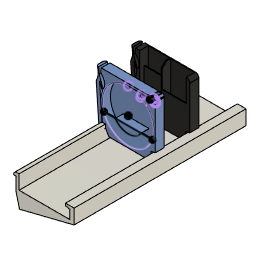
SMD Cassette System v11 (Autodesk Fusion 360 design; units mm, degrees)
Autodesk Fusion 360 part; units mm, degrees
note: some values were not read from the file. Set by a fixed rule: which face or edge a step refers to.
sketch "Base Shape" plane through (0, 0, 0) normal (0, 1, 0) x (1, 0, 0)
  line L0 (5, -7) -> (5, -11)
  line L1 (5, -11) -> (0, -11)
  line L2 (0, -65) -> (0, -11)
  line L3 (63, -65) -> (0, -65)
  line L4 (63, -11) -> (63, -65)
  line L5 (58, -10.01) -> (63, -11)
  line L6 (58, -4.99) -> (58, -10.01)
  line L7 (63, -4) -> (58, -4.99)
  line L8 (9, 0) -> (5, -7)
  line L9 (59.0007, 0) -> (9, 0)
  line L10 (63, -7.5) -> (58, -7.5) construction
  arc A0 (63, -4) -> (59.0007, 0) centre (59.0007, -3.9993) ccw
  line L11 (0, -1.75) -> (0, -22.5) construction
  line L12 (1.75, 0) -> (22.5, 0) construction
  line L13 (0.3, -10.5) -> (4.5, -10.5)
  line L14 (4.5, -10.5) -> (4.5, 6)
  line L15 (4.5, 6) -> (63.5, 6)
  line L16 (63.5, 6) -> (63.5, -4.41)
  line L17 (63.5, -4.41) -> (58.5, -5.4)
  line L18 (58.5, -5.4) -> (58.5, -8)
  line L19 (68.5, -8) -> (68.5, 9)
  line L20 (68.5, 9) -> (4.9505, 24.8447)
  line L21 (1, 9) -> (1, -6.5)
  line L22 (-1.7, -8.5) -> (-1.7, -6.5)
  line L23 (1, -6.5) -> (-1.7, -6.5)
  line L24 (68.5, 9) -> (1, 9)
  line L25 (1, 9) -> (4.9505, 24.8447)
  line L26 (0.3, -10.5) -> (-1.7, -8.5)
  line L27 (58.5, -8) -> (68.5, -8)
  line L28 (0.3, -10.5) -> (0.3, -8.5) construction
  line L29 (0.3, -8.5) -> (-1.7, -8.5) construction
  line L30 (31.5, -65) -> (31.5, 6) construction
  dimension "d139" = 4
  dimension "d140" = 7
  dimension "d141" = 65
  dimension "d142" = 63
  dimension "d144" = 4
  dimension "d168" = 7
  dimension "d216" = 3.5
  dimension "d217" = 4
  dimension "d224" = 6
  dimension "d226" = 5
  dimension "d227" = 3
  dimension "d228" = 14
  dimension "d283" = 6.2
  dimension "d284" = 2
  dimension "d344" = 10
  dimension "d348" = 2.6
  dimension "d352" = 59
  dimension "d353" = 8
  dimension "d355" = 10.5
  dimension "d356" = 5
  dimension "d357" = 5
  dimension "d358" = 27
  dimension "d359" = 11.2
  dimension "d360" = 0.5
  constraint perpendicular L3 L4
  constraint perpendicular L0 L1
  constraint parallel L4 L6
  constraint horizontal L9
  constraint perpendicular L1 L2
  constraint perpendicular L4 L10
  constraint symmetric L5 L7 L10
  constraint coincident L9 A0.end
  constraint tangent L9 A0
  constraint coincident L7.start A0.start
  constraint coincident L9.start A0.end
  constraint collinear L2 L11
  constraint collinear L9 L12
  constraint equal L5 L7
  constraint perpendicular L11 L13
  constraint perpendicular L13 L14
  constraint perpendicular L14 L15
  constraint perpendicular L15 L16
  constraint perpendicular L15 L18
  constraint perpendicular L13 L22
  constraint perpendicular L22 L23
  constraint parallel L7 L17
  constraint coincident L21 L24.end
  constraint perpendicular L21 L24
  constraint coincident L21.start L24.end
  constraint perpendicular L20 L25
  constraint coincident L13 L26.start
  constraint coincident L22 L26.end
  constraint coincident L13.start L26.start
  constraint coincident L22.start L26.end
  constraint perpendicular L19 L27
  constraint tangent L4 A0
  constraint horizontal L29
  constraint vertical L28
  constraint equal L28 L29
  constraint midpoint L3 L30.start
  constraint coincident L15 L30.end
  constraint vertical L30
  constraint midpoint L6 L10.end
  constraint coincident L4 L10.start
  measures "d139" distance of L0.start L0.end
  measures "d140" vertical distance of L0.start L8.start
  measures "d141" distance of L3 L9
  measures "d142" distance of L2 L4
  measures "d144" horizontal distance of L0.start L8.start
  measures "d168" vertical distance of L4.start L7.start
  measures "d216" distance of L14 L21
  measures "d217" distance of L13 L23
  measures "d224" distance of L9 L15
  measures "d226" distance of L16 L19
  measures "d227" distance of L15 L24
  measures "d228" angle of L20 L24
  measures "d283" distance of L14 L22
  measures "d284" distance of L22 L13.start
  measures "d344" distance of L18 L19
  measures "d348" distance of L17.end L18.end
  measures "d352" distance of L14 L16
  measures "d353" distance of L12 L27
  measures "d355" distance of L12 L13
  measures "d356" distance of L0 L2
  measures "d357" distance of L4 L6
  measures "d358" distance of L14 L30
  measures "d359" angle of L17 L27
  measures "d360" distance of L10 L27
sketch "Geometry Outline" plane through (0, 0, 0) normal (0, 1, 0) x (-1, 0, 0) in component "Cassette"
  circle A0 centre (-31.5, 32.5) radius 30
  line L0 (-63, 11) -> (-63, 65) construction
  line L1 (-63, 65) -> (0, 65) construction
  line L2 (-31.5, 62.5) -> (-63, 62.5)
  line L3 (-63, 61.4) -> (-47.0399, 61.4)
  line L4 (-54.8759, 62.5) -> (-57.8759, 65)
  arc A1 (-61, 65) -> (-63, 63) centre (-61, 63) ccw
  arc A2 (-46.3, 58.5952) -> (-47.0399, 61.4) centre (-47.0399, 59.9) ccw
  line L5 (0, 65) -> (0, 11) construction
  circle A3 centre (0, 49) radius 16 construction
  line L6 (5.9573, 52.413) -> (2.3229, 0.439)
  line L7 (2.3229, 0.439) -> (-0.3073, 0.623)
  line L8 (-0.3073, 0.623) -> (-4.2973, 6.1147)
  line L9 (-4.2973, 6.1147) -> (-1.3046, 5.9054)
  line L10 (-1.3046, 5.9054) -> (2.8103, 64.7513)
  circle A4 centre (-31.5, 32.5) radius 31.5
  line L11 (2.8103, 64.7513) -> (6.0319, 64.526)
  line L12 (-0.0767, 30.3027) -> (-1.4265, 11)
  line L13 (6.4518, 59.4844) -> (22.4128, 58.3683) construction
  arc A5 (6.0319, 64.526) -> (5.9573, 52.413) centre (22.4128, 58.3683) ccw
  line L14 (-5, 7) -> (-5, 11)
  line L15 (-9, 0) -> (-5, 7)
  line L16 (-59.0007, 0) -> (-9, 0)
  arc A6 (-63, 4) -> (-59.0007, 0) centre (-59.0007, 3.9993) ccw
  line L17 (-63, 4) -> (-58, 4.99)
  line L18 (-58, 4.99) -> (-58, 10.01)
  line L19 (-58, 10.01) -> (-63, 11)
  line L20 (-63, 11) -> (-63, 61.4)
  line L21 (-57.8759, 65) -> (0, 65)
  line L22 (0, 65) -> (0.5716, 60.0328)
  line L23 (0.5716, 60.0328) -> (-6.4766, 51.6332)
  line L24 (-1.5649, 42.3051) -> (1.9557, 52.5297)
  line L25 (-2.3288, 44.3867) -> (2.333, 57.9257)
  line L26 (-5, 11) -> (-1.4265, 11)
  line L27 (-1.9368, 43.3751) -> (2.1444, 55.2277) construction
  line L28 (0.1038, 49.3014) -> (3.6495, 48.0805) construction
  line L29 (0, 65) -> (1.8766, 48.691) construction
  line L30 (3.7977, 50.1996) -> (2.3436, 29.4054) construction
  circle A7 centre (0, 49) radius 49 construction
  line L31 (-57.8759, 65) -> (-61, 65)
  line L32 (-63, 63) -> (-63, 61.4)
  line L33 (-61, 65) -> (-58, 62.5)
  point P0 (-63, 65)
  point P1 (0, 65)
  point P2 (1.8766, 48.691)
  point P3 (0.1038, 49.3014)
  dimension "d151" = 60
  dimension "d153" = 32.5
  dimension "d154" = 1.1
  dimension "d156" = 3
  dimension "d169" = 2
  dimension "d183" = 16
  dimension "d184" = 3
  dimension "d185" = 4
  dimension "d188" = 5.2
  dimension "d190" = 50
  dimension "d193" = 4
  dimension "d196" = 5
  dimension "d197" = 16
  dimension "d198" = 17.5
  dimension "d200" = 31.5
  dimension "d205" = 50
  dimension "d206" = 5
  dimension "d208" = 15
  dimension "d209" = 1.4
  dimension "d214" = 3.75
  dimension "d215" = 0.6
  dimension "d327" = 1.5
  dimension "d328" = 2
  constraint coincident A0 L2.start
  constraint coincident L0 L2.end
  constraint tangent A0 L2
  constraint perpendicular L0 L2
  constraint coincident L0 L3.start
  constraint perpendicular L0 L3
  constraint coincident L2 L4.start
  constraint coincident L1 L4.end
  constraint coincident L1 A1.start
  constraint coincident L0 A1.end
  constraint tangent L1 A1
  constraint tangent L0 A1
  constraint coincident A0 A2.start
  constraint tangent L3 A2
  constraint tangent A0 A2
  constraint coincident L5 A3.centre
  constraint coincident P1 A3
  constraint perpendicular L6 L7
  constraint perpendicular L6 L9
  constraint perpendicular L9 L10
  constraint concentric A0 A4
  constraint coincident A3 L10.end
  constraint tangent L5 A4
  constraint coincident A4 L12.start
  constraint tangent A4 L12
  constraint parallel L10 L12
  constraint coincident L6 L13.start
  constraint perpendicular L6 L13
  constraint coincident L6 A5.end
  constraint coincident L13.end A5.centre
  constraint coincident L11 A5.start
  constraint coincident L11.end A5.start
  constraint coincident L6.start A5.end
  constraint coincident L0.start L19.end
  constraint coincident P1 L1.end
  constraint coincident A4 L23.end
  constraint coincident A4 L24.start
  constraint coincident L10 L24.end
  constraint coincident A4 L25.start
  constraint coincident L10 L25.end
  constraint coincident L14.end L26.start
  constraint horizontal L26
  constraint parallel L24 L25
  constraint coincident A4 L27.start
  constraint coincident L10 L27.end
  constraint parallel L24 L27
  constraint coincident L27 P3
  constraint perpendicular L24 L28
  constraint midpoint L28 P2
  constraint coincident P2 L29.end
  constraint collinear L22 L29
  constraint midpoint L27 P3
  constraint coincident A3.centre L27
  constraint parallel L6 L30
  constraint coincident L28.end L30
  constraint concentric A3 A7
  constraint coincident origin A7
  constraint coincident L2 L33.end
  constraint parallel L4 L33
  constraint coincident A1.start L31.end
  measures "d151" diameter of A0
  measures "d153" distance of A0.centre L1
  measures "d154" distance of L2 L3
  measures "d156" horizontal distance of L4.start L4.end
  measures "d169" radius of A1
  measures "d183" distance of A3.centre P1
  measures "d184" distance of L8.end L9.end
  measures "d185" distance of L6 L10
  measures "d188" distance of L7 L9
  measures "d190" angle of L8 L9
  measures "d193" angle of L5 L10
  measures "d196" distance of L11 L13
  measures "d197" distance of L13.start L13.end
  measures "d198" radius of A5
  measures "d200" distance of L0 A0.centre
  measures "d205" angle of L21 L23
  measures "d206" distance of P1 L22.end
  measures "d208" angle of L10 L27
  measures "d209" distance of L24 L25
  measures "d214" distance of P3 L28.end
  measures "d215" distance of origin L7
  measures "d327" radius of A2
  measures "d328" distance of L4 L33
extrude "Extrude12" add sketch "Geometry Outline" along normal blind 10.2 makes body 1 in component "Cassette"
extrude "Extrude13" cut sketch "Geometry Outline" along normal up to surface (9.3 mm away) contours A0 | A0 L2 A2 A4 | L2 L3 A2 A4 L32 | L2 L4 L31 L33 picked at (-41.0262, 61.4298) bodies 1 in component "Cassette"
sketch "Lip" plane through (0, 0, 0) normal (0, -1, 0) x (1, 0, 0) in component "Cassette"
  arc A0 (31.5, 62.5) -> (46.3, 58.5952) centre (31.5, 32.5) ccw
  line L0 (61, 65) -> (58, 62.5)
  line L1 (58, 62.5) -> (63, 62.5)
  line L2 (63, 61.4) -> (47.0399, 61.4)
  line L3 (63, 62.5) -> (63, 61.4)
  line L4 (58, 62.5) -> (56.68, 61.4)
  line L5 (3.2157, 22.5) -> (59.7843, 22.5)
  arc A1 (16.5334, 22.5) -> (46.4666, 22.5) centre (31.5, 32.5) ccw
  dimension "d333" = 10
  dimension "d336" = 12
  constraint coincident L0.end L1.start
  constraint coincident L2 L4.end
  constraint collinear L0 L4
  constraint coincident A0 L5.start
  constraint coincident A0 L5.end
  constraint horizontal L5
  constraint coincident L5 A1.start
  constraint coincident A0.centre A1.centre
  constraint coincident L5 A1.end
  measures "d333" distance of A0.centre L5
  measures "d336" distance of A0 A1
extrude "Extrude14" add sketch "Lip" against normal blind 0.9 bodies 1 in component "Cassette"
chamfer "Chamfer2" distance 1.5 distance2 2 2 edges at (-4.9132, 10.2, 58.4761) (-4.9132, 0, 58.4761) measured on face at (42.4922, 10.2, 41.5477) measured on face at (40.9281, 0, 14.5033) on bodies 1 in component "Cassette"
fillet "Fillet9" radius 3 1 edges at (-0.5716, 5.1, 60.0328) on bodies 1 in component "Cassette"
fillet "Fillet9" radius 11 1 edges at (6.4766, 5.1, 51.6332) on bodies 1 in component "Cassette"
fillet "Fillet9" radius 0.25 2 edges at (2.3288, 5.1, 44.3867) (-1.9557, 5.1, 52.5297) on bodies 1 in component "Cassette"
fillet "Fillet9" radius 1.5 2 edges at (-2.333, 5.1, 57.9257) (1.5649, 5.1, 42.3051) on bodies 1 in component "Cassette"
fillet "Fillet10" radius 0.5 2 edges at (57.8759, 4.65, 65) (61, 4.65, 65) on bodies 1 in component "Cassette"
fillet "Fillet11" radius 3 2 edges at (54.8759, 4.65, 62.5) (56.68, 0.45, 61.4) on bodies 1 in component "Cassette"
fillet "Fillet12" radius 1 3 edges at (-2.3229, 5.1, 0.439) (0.3073, 5.1, 0.623) (9, 5.1, 0) on bodies 1 in component "Cassette"
extrude "Extrude15" add sketch "Lip" against normal up to surface (9.3 mm away) contours L5 A1 bodies 1 in component "Cassette"
extrude "Extrude1" add sketch "Base Shape" along normal mid plane 200 separate body contours L13 L14 L15 L16 L17 L18 L19 L21 L22 L23 L24 L26 L27 | L20 L24 L25 makes body 2 in component "OG Rail"
ref_plane "WorkPlane1" through (33.4, 96.4, -7.1723) normal (0, 1, 0) x (0, 0, 1) in component "OG Rail"
sketch "Compartment Profile" plane through (33.4, 96.4, -7.1723) normal (0, 1, 0) x (1, 0, 0) in component "OG Rail"
  line L0 (35.1, 1.8277) -> (-32.4, 1.8277) construction
  line L1 (-32.4, 1.8277) -> (-28.4495, 17.6723) construction
  line L2 (35.1, 1.8277) -> (-28.4495, 17.6723) construction
  line L3 (19.6782, 4.0238) -> (-28.8366, 16.1199)
  arc A0 (19.4086, 1.8277) -> (19.6782, 4.0238) centre (19.4086, 2.9423) ccw
  line L4 (-28.4495, 17.6723) -> (-32.4, 1.8277)
  line L5 (-32.4, 1.8277) -> (19.4086, 1.8277)
  dimension "d279" = 50
  dimension "d282" = 1.6
  constraint tangent L3 A0
  constraint coincident L3 A0.end
  constraint parallel L2 L3
  constraint coincident L0 A0.start
  constraint tangent L0 A0
  constraint coincident L1 L3.end
  constraint coincident L3.start A0.end
  constraint coincident L0.end L1.start
  measures "d279" distance of L1 L3.start
  measures "d282" distance of L2 L3
extrude "Extrude3" cut sketch "Compartment Profile" against normal up to surface (192.8 mm away) bodies 2 in component "OG Rail"
extrude "Extrude2" add 1 faces at (19.4573, 96.4, -13.7641) along direction (0, 1, 0) blind 1.8 separate body on bodies 2 makes body 3 in component "OG Rail"
pattern_linear "R-Pattern2" count 4 spacing 64.8667 along (0, -1, 0) of bodies 3 makes body 4 at (19.4573, 31.5333, -13.7641) makes body 5 at (19.4573, -33.3333, -13.7641) makes body 6 at (19.4573, -98.2, -13.7641) in component "OG Rail"
combine "Combine1" operation add target body 2 tool bodies 3 4 6 5 in component "OG Rail"
sketch "Lid outline" plane through (-1.1711, 0, -0.292) normal (-0.970296, 0, -0.241922) x (0, -1, 0) in component "Lid"
  line L0 (100, -8.9746) -> (96.4, -8.9746)
  line L1 (96.4, -8.9746) -> (96.4, -23.7043)
  line L2 (96.4, -23.7043) -> (33.3333, -23.7043)
  line L3 (33.3333, -23.7043) -> (33.3333, -8.9746)
  line L4 (33.3333, -8.9746) -> (31.5333, -8.9746)
  line L5 (31.5333, -8.9746) -> (31.5333, -23.7043)
  line L6 (31.5333, -23.7043) -> (-31.5333, -23.7043)
  line L7 (-31.5333, -23.7043) -> (-31.5333, -8.9746)
  line L8 (-31.5333, -8.9746) -> (-33.3333, -8.9746)
  line L9 (-33.3333, -8.9746) -> (-33.3333, -23.7043)
  line L10 (-33.3333, -23.7043) -> (-96.4, -23.7043)
  line L11 (-96.4, -23.7043) -> (-96.4, -8.9746)
  line L12 (-96.4, -8.9746) -> (-100, -8.9746)
  line L13 (-100, -8.9746) -> (-100, -25.3043)
  line L14 (-100, -25.3043) -> (100, -25.3043)
  line L15 (100, -25.3043) -> (100, -8.9746)
  line L16 (-100, -25.3043) -> (-100, -8.9746)
  line L17 (100, -25.3043) -> (-100, -25.3043)
  line L18 (100, -8.9746) -> (100, -25.3043)
  line L19 (100, 6.065) -> (100, -8.9746)
  line L20 (-100, -8.9746) -> (-100, 6.065)
  line L21 (-99, -24.5043) -> (99, -24.5043)
  line L22 (99, -24.5043) -> (99, -7.9746)
  line L23 (99, -7.9746) -> (-99, -7.9746)
  line L24 (-99, -7.9746) -> (-99, -24.5043)
  line L25 (-33.3333, -8.9746) -> (-96.4, -8.9746)
  dimension "d286" = 1
  dimension "d287" = 0.8
  dimension "d288" = 1
  dimension "d289" = 1
  constraint horizontal L21
  constraint vertical L22
  constraint horizontal L23
  constraint vertical L24
  measures "d286" distance of L16 L24
  measures "d287" distance of L17 L21
  measures "d288" distance of L15 L22
  measures "d289" distance of L23 L25
extrude "Extrude4" cut sketch "Lid outline" against normal blind 1.2 contours L0 L1 L2 L3 L4 L5 L6 L7 L8 L9 L10 L11 L12 L21 L22 L24 | L0 L1 L2 L3 L4 L5 L6 L7 L8 L12 L22 L23 L24 L25 | L9 L10 L11 L25 bodies 2 in component "OG Rail"
extrude "Extrude1'" add sketch "Lid outline" against normal up to surface (1.4 mm away) separate body contours L0 L1 L2 L3 L4 L5 L6 L7 L8 L9 L10 L11 L12 L21 L22 L24 | L0 L1 L2 L3 L4 L5 L6 L7 L8 L12 L22 L23 L24 L25 | L9 L10 L11 L25 makes body 7 in component "Lid"
move_face "OffsetFaces1" offset -0.2 6 faces at (1.825, 99, -8.4508) (4.4103, 99, -18.8198) (1.2109, -33, -7.9168) (3.1579, -99, -13.797) (1.7443, -99, -8.1273) (5.2098, 33, -23.9555) on bodies 7 in component "Lid"
sketch "Lid Trim Cut" plane through (0, -100, 0) normal (0, -1, 0) x (1, 0, 0) in component "Lid"
  line L0 (4.5, -6) -> (4.5, 10.5)
  line L1 (4.5, 10.5) -> (0.3, 10.5)
  line L2 (0.3, 10.5) -> (-1.7, 8.5)
  line L3 (-1.7, 8.5) -> (-1.7, 6.5)
  line L4 (-1.7, 6.5) -> (1, 6.5)
  line L5 (1, 6.5) -> (1, -9)
  line L6 (1, -9) -> (4.9505, -24.8447)
  line L7 (4.9505, -24.8447) -> (68.5, -9)
  line L8 (68.5, -9) -> (68.5, 8)
  line L9 (58.5, 8) -> (58.5, 5.4)
  line L10 (58.5, 5.4) -> (63.5, 4.41)
  line L11 (63.5, 4.41) -> (63.5, -6)
  line L12 (63.5, -6) -> (4.5, -6)
  line L13 (1, -9) -> (1, 6.5)
  line L14 (-2.6384, 5.5928) -> (1, -9)
  line L15 (1, 6.5) -> (-2.6384, 5.5928)
  line L16 (68.5, 8) -> (58.5, 8)
  constraint coincident L5.end L6.start
  constraint coincident L4.end L5.start
  constraint coincident L14.start L15.end
extrude "Extrude2'" cut sketch "Lid Trim Cut" against normal up to surface (200 mm away) contours L5 L13 L14 L15 bodies 7 in component "Lid"
sketch "Geometry Outline (2)" plane through (0, 0, 0) normal (0, 1, 0) x (-1, 0, 0) in component "Misc Cassette"
  line L0 (-63, 11) -> (-63, 65) construction
  line L1 (-63, 65) -> (0, 65) construction
  arc A0 (-59, 65) -> (-63, 61) centre (-59, 61) ccw
  line L2 (0, 65) -> (0, 11) construction
  circle A1 centre (0, 49) radius 16 construction
  line L3 (5.9573, 52.413) -> (2.3229, 0.439)
  line L4 (2.3229, 0.439) -> (-0.3073, 0.623)
  line L5 (-0.3073, 0.623) -> (-4.2973, 6.1147)
  line L6 (-4.2973, 6.1147) -> (-1.3046, 5.9054)
  line L7 (-1.3046, 5.9054) -> (2.8103, 64.7513)
  circle A2 centre (-31.5, 32.5) radius 31.5
  line L8 (2.8103, 64.7513) -> (6.0319, 64.526)
  line L9 (-0.0767, 30.3027) -> (-1.4265, 11)
  line L10 (6.4518, 59.4844) -> (22.4128, 58.3683) construction
  arc A3 (6.0319, 64.526) -> (5.9573, 52.413) centre (22.4128, 58.3683) ccw
  line L11 (-5, 7) -> (-5, 11)
  line L12 (-9, 0) -> (-5, 7)
  line L13 (-59.0007, 0) -> (-9, 0)
  arc A4 (-63, 4) -> (-59.0007, 0) centre (-59.0007, 3.9993) ccw
  line L14 (-63, 4) -> (-58, 4.99)
  line L15 (-58, 4.99) -> (-58, 10.01)
  line L16 (-58, 10.01) -> (-63, 11)
  line L17 (-63, 11) -> (-63, 60.5)
  line L18 (-59, 65) -> (0, 65)
  line L19 (0, 65) -> (0.5716, 60.0328)
  line L20 (0.5716, 60.0328) -> (-6.4766, 51.6332)
  line L21 (-1.5649, 42.3051) -> (1.9557, 52.5297)
  line L22 (-2.3288, 44.3867) -> (2.333, 57.9257)
  line L23 (-5, 11) -> (-1.4265, 11)
  line L24 (-1.9368, 43.3751) -> (2.1444, 55.2277) construction
  line L25 (0.1038, 49.3014) -> (3.6495, 48.0805) construction
  line L26 (0, 65) -> (1.8766, 48.691) construction
  line L27 (3.7977, 50.1996) -> (2.3436, 29.4054) construction
  circle A5 centre (0, 49) radius 49 construction
  line L28 (-63, 61) -> (-63, 60.5)
  point P0 (-63, 65)
  point P1 (0, 65)
  point P2 (1.8766, 48.691)
  point P3 (0.1038, 49.3014)
  dimension "d153_1" = 32.5
  dimension "d169_1" = 4
  dimension "d183_1" = 16
  dimension "d184_1" = 3
  dimension "d185_1" = 4
  dimension "d188_1" = 5.2
  dimension "d190_1" = 50
  dimension "d193_1" = 4
  dimension "d196_1" = 5
  dimension "d197_1" = 16
  dimension "d198_1" = 17.5
  dimension "d200_1" = 31.5
  dimension "d205_1" = 50
  dimension "d206_1" = 5
  dimension "d208_1" = 15
  dimension "d209_1" = 1.4
  dimension "d214_1" = 3.75
  dimension "d215_1" = 0.6
  constraint coincident L0 L17.end
  constraint coincident L1 A0.start
  constraint coincident L0 A0.end
  constraint tangent L1 A0
  constraint tangent L0 A0
  constraint coincident L2 A1.centre
  constraint coincident P1 A1
  constraint perpendicular L3 L4
  constraint perpendicular L3 L6
  constraint perpendicular L6 L7
  constraint coincident A1 L7.end
  constraint tangent L2 A2
  constraint coincident A2 L9.start
  constraint tangent A2 L9
  constraint parallel L7 L9
  constraint coincident L3 L10.start
  constraint perpendicular L3 L10
  constraint coincident L3 A3.end
  constraint coincident L10.end A3.centre
  constraint coincident L8 A3.start
  constraint coincident L8.end A3.start
  constraint coincident L3.start A3.end
  constraint coincident L0.start L16.end
  constraint coincident P1 L1.end
  constraint coincident A2 L20.end
  constraint coincident A2 L21.start
  constraint coincident L7 L21.end
  constraint coincident A2 L22.start
  constraint coincident L7 L22.end
  constraint coincident L11.end L23.start
  constraint horizontal L23
  constraint parallel L21 L22
  constraint coincident A2 L24.start
  constraint coincident L7 L24.end
  constraint parallel L21 L24
  constraint coincident L24 P3
  constraint perpendicular L21 L25
  constraint midpoint L25 P2
  constraint coincident P2 L26.end
  constraint collinear L19 L26
  constraint midpoint L24 P3
  constraint coincident A1.centre L24
  constraint parallel L3 L27
  constraint coincident L25.end L27
  constraint concentric A1 A5
  constraint coincident origin A5
  constraint coincident A0.start L18.start
  measures "d153_1" distance of L1 A2.centre
  measures "d169_1" radius of A0
  measures "d183_1" distance of A1.centre P1
  measures "d184_1" distance of L5.end L6.end
  measures "d185_1" distance of L3 L7
  measures "d188_1" distance of L4 L6
  measures "d190_1" angle of L5 L6
  measures "d193_1" angle of L2 L7
  measures "d196_1" distance of L8 L10
  measures "d197_1" distance of L10.start L10.end
  measures "d198_1" radius of A3
  measures "d200_1" distance of L0 A2.centre
  measures "d205_1" angle of L18 L20
  measures "d206_1" distance of P1 L19.end
  measures "d208_1" angle of L7 L24
  measures "d209_1" distance of L21 L22
  measures "d214_1" distance of P3 L25.end
  measures "d215_1" distance of origin L4
extrude "Extrude12'" add sketch "Geometry Outline (2)" along normal blind 10.7 separate body makes body 8 in component "Misc Cassette"
chamfer "Chamfer2'" distance 1.5 distance2 2 2 edges at (-4.9132, 10.7, 58.4761) (-4.9132, 0, 58.4761) measured on face at (42.8255, 10.7, 49.7111) measured on face at (42.8255, 0, 49.7111) on bodies 8 in component "Misc Cassette"
fillet "Fillet10'" radius 3 1 edges at (-0.5716, 5.35, 60.0328) on bodies 8 in component "Misc Cassette"
fillet "Fillet11'" radius 11 1 edges at (6.4766, 5.35, 51.6332) on bodies 8 in component "Misc Cassette"
fillet "Fillet12'" radius 0.25 2 edges at (2.3288, 5.35, 44.3867) (-1.9557, 5.35, 52.5297) on bodies 8 in component "Misc Cassette"
fillet "Fillet13" radius 1.5 2 edges at (1.5649, 5.35, 42.3051) (-2.333, 5.35, 57.9257) on bodies 8 in component "Misc Cassette"
sketch "Slots" plane through (0, 0, 65) normal (0, 0, 1) x (-1, 0, 0) in component "Misc Cassette"
  line L0 (0, 0) -> (-59, 0)
  line L1 (-59, 0) -> (-59, -10.7)
  line L2 (-59, -10.7) -> (0, -10.7)
  line L3 (0, -10.7) -> (0, 0)
  line L4 (-63, 0) -> (-59, 0)
  line L5 (-63, 0) -> (-63, -10.7)
  line L6 (-63, -10.7) -> (-59, -10.7)
  line L7 (-59, -10.7) -> (-59, 0)
  line L8 (-29.9243, -0.9) -> (-4.9243, -0.9)
  line L9 (-4.9243, -0.9) -> (-4.9243, -4.9)
  line L10 (-4.9243, -4.9) -> (-29.9243, -4.9)
  line L11 (-29.9243, -4.9) -> (-29.9243, -0.9)
  line L12 (-29.9243, -5.8) -> (-4.9243, -5.8)
  line L13 (-4.9243, -5.8) -> (-4.9243, -9.8)
  line L14 (-4.9243, -9.8) -> (-29.9243, -9.8)
  line L15 (-29.9243, -9.8) -> (-29.9243, -5.8)
  line L16 (-20.4907, 0) -> (-20.4907, -0.9) construction
  line L17 (-20.4907, -4.9) -> (-20.4907, -5.8) construction
  line L18 (-20.4907, -9.8) -> (-20.4907, -10.7) construction
  line L19 (-1.4508, 0) -> (-4.0243, 0) construction
  line L20 (-1.4508, 0) -> (-1.4508, -10.7) construction
  line L21 (-4.0243, -10.7) -> (-1.4508, -10.7) construction
  line L22 (-2.9827, -10.7) -> (-2.9827, 0) construction
  line L23 (-31.1243, -9.8) -> (-62.1, -9.8)
  line L24 (-62.1, -9.8) -> (-62.1, -0.9)
  line L25 (-62.1, -0.9) -> (-31.1243, -0.9)
  line L26 (-31.1243, -0.9) -> (-31.1243, -9.8)
  line L27 (-62.1, -8.0888) -> (-63, -8.0888) construction
  line L28 (-4.0243, 0) -> (-4.0243, -10.7) construction
  line L29 (-4.9243, -8.157) -> (-4.0243, -8.157) construction
  dimension "d305" = 0.9
  dimension "d306" = 25
  dimension "d317" = 1.2
  constraint horizontal L8
  constraint vertical L9
  constraint horizontal L10
  constraint vertical L11
  constraint horizontal L12
  constraint horizontal L14
  constraint collinear L11 L15
  constraint collinear L9 L13
  constraint coincident L0 L16.start
  constraint coincident L8 L16.end
  constraint perpendicular L0 L16
  constraint coincident L10 L17.start
  constraint coincident L12 L17.end
  constraint perpendicular L12 L17
  constraint coincident L14 L18.start
  constraint coincident L2 L18.end
  constraint perpendicular L2 L18
  constraint equal L17 L18
  constraint equal L16 L17
  constraint equal L11 L15
  constraint horizontal L23
  constraint vertical L24
  constraint horizontal L25
  constraint vertical L26
  constraint collinear L14 L23
  constraint collinear L8 L25
  constraint coincident L24 L27.start
  constraint coincident L5 L27.end
  constraint perpendicular L5 L27
  constraint equal L18 L27
  constraint coincident L19.end L28.start
  constraint coincident L21.start L28.end
  constraint coincident L13 L29.start
  constraint coincident L28 L29.end
  constraint perpendicular L28 L29
  constraint equal L27 L29
  measures "d305" distance of L16.start L16.end
  measures "d306" distance of L8.start L8.end
  measures "d317" distance of L15 L26
extrude "Extrude15'" cut sketch "Slots" against normal up to surface (53.1 mm away) contours L1 L7 L23 L25 L26 | L8 L9 L10 L11 | L12 L13 L14 L15 bodies 8 in component "Misc Cassette"
sketch "Stairs" plane through (0, 0, 0) normal (0, -1, 0) x (1, 0, 0) in component "Misc Cassette"
  arc A0 (-0.424, 61.3152) -> (0.2582, 59.0439) centre (2.5563, 60.9723) ccw
  line L0 (0.2582, 59.0439) -> (1.4508, 57.6226)
  arc A1 (2.9827, 45.8797) -> (1.4508, 57.6226) centre (-6.9757, 50.5519) ccw
  arc A2 (2.9827, 45.8797) -> (2.5814, 44.9885) centre (31.5, 32.5) ccw
  arc A3 (2.1155, 45.0063) -> (2.5814, 44.9885) centre (2.3519, 45.0877) ccw
  line L1 (2.1155, 45.0063) -> (-2.2687, 57.739)
  arc A4 (-2.3468, 58.1227) -> (-2.2687, 57.739) centre (-0.8505, 58.2273) ccw
  line L2 (-2.3468, 58.1227) -> (-2.8103, 64.7513)
  line L3 (-2.8103, 64.7513) -> (-4.476, 64.6348)
  arc A5 (-5.737, 49.2624) -> (-4.476, 64.6348) centre (-22.4128, 58.3683) ccw
  line L4 (-5.737, 49.2624) -> (-2.3229, 0.439)
  line L5 (-2.3229, 0.439) -> (0.3073, 0.623)
  line L6 (0.3073, 0.623) -> (4.2973, 6.1147)
  line L7 (4.2973, 6.1147) -> (1.3046, 5.9054)
  line L8 (1.3046, 5.9054) -> (-1.8232, 50.6354)
  arc A6 (-1.3375, 50.7342) -> (-1.8232, 50.6354) centre (-1.5739, 50.6528) ccw
  line L9 (-1.3375, 50.7342) -> (1.403, 42.7754)
  arc A7 (1.4172, 41.8422) -> (1.403, 42.7754) centre (-0.0153, 42.287) ccw
  arc A8 (1.4172, 41.8422) -> (0.0767, 30.3027) centre (31.5, 32.5) ccw
  line L10 (0.0767, 30.3027) -> (1.4265, 11)
  line L11 (1.4265, 11) -> (5, 11)
  line L12 (5, 11) -> (5, 7)
  line L13 (5, 7) -> (9, 0)
  line L14 (9, 0) -> (59.0007, 0)
  arc A9 (59.0007, 0) -> (63, 4) centre (59.0007, 3.9993) ccw
  line L15 (63, 4) -> (58, 4.99)
  line L16 (58, 4.99) -> (58, 10.01)
  line L17 (58, 10.01) -> (63, 11)
  line L18 (63, 11) -> (63, 61)
  arc A10 (63, 61) -> (59, 65) centre (59, 61) ccw
  line L19 (59, 65) -> (0, 65)
  line L20 (0, 65) -> (-0.424, 61.3152)
  line L21 (4.9243, 11.9) -> (29.9243, 11.9)
  line L22 (29.9243, 11.9) -> (29.9243, 65)
  line L23 (29.9243, 65) -> (4.9243, 65)
  line L24 (4.9243, 65) -> (4.9243, 11.9)
  line L25 (31.1243, 11.9) -> (59, 11.9)
  line L26 (59, 11.9) -> (59, 65)
  line L27 (59, 65) -> (31.1243, 65)
  line L28 (31.1243, 65) -> (31.1243, 11.9)
  line L29 (29.9243, 65) -> (31.1243, 65)
  line L30 (29.9243, 11.9) -> (31.1243, 11.9)
  line L31 (4.9243, 47.3) -> (29.9243, 47.3)
  line L32 (4.9243, 29.6) -> (29.9243, 29.6)
  line L33 (31.1243, 38.45) -> (59, 38.45)
  line L34 (19.4881, 65) -> (19.4881, 47.3) construction
  line L35 (19.4881, 47.3) -> (19.4881, 29.6) construction
  line L36 (19.4881, 29.6) -> (19.4881, 11.9) construction
  constraint coincident L22.end L23.start
  constraint coincident L27.end L28.start
  constraint coincident L21.end L22.start
  constraint coincident L25.start L28.end
  constraint coincident L24 L31.start
  constraint coincident L22 L31.end
  constraint perpendicular L22 L31
  constraint coincident L24 L32.start
  constraint coincident L22 L32.end
  constraint perpendicular L22 L32
  constraint coincident L26 L33.end
  constraint midpoint L28 L33.start
  constraint midpoint L26 L33.end
  constraint coincident L23 L34.start
  constraint coincident L31 L34.end
  constraint perpendicular L31 L34
  constraint coincident L32 L35.end
  constraint perpendicular L32 L35
  constraint coincident L21 L36.end
  constraint perpendicular L21 L36
  constraint equal L34 L35
  constraint equal L35 L36
extrude "Extrude16" cut sketch "Stairs" against normal up to surface (0.9 mm away) contours L19 L26 L27 L28 L33 bodies 8 in component "Misc Cassette"
extrude "Extrude17" cut sketch "Stairs" against normal up to surface (5.8 mm away) contours L19 L22 L23 L24 L31 bodies 8 in component "Misc Cassette"
extrude "Extrude18" cut sketch "Stairs" against normal up to surface (0.9 mm away) contours L22 L24 L31 L32 bodies 8 in component "Misc Cassette"
chamfer "Chamfer3" distance 5 angle 45 1 edges at (30.5243, 0, 65) on bodies 8 in component "Misc Cassette"
component "Cassette" placed x (1, 0, 0) y (0, 1, 0) z (0, 0, 1) at (0, 0, 0)
component "OG Rail" placed x (1, 0, 0) y (0, 1, 0) z (0, 0, 1) at (0, 0, 0)
component "Misc Cassette" placed x (1, 0, 0) y (0, 1, 0) z (0, 0, 1) at (0, 40, 0)
component "Lid" placed x (1, 0, 0) y (0, 1, 0) z (0, 0, 1) at (0, 0, 0) in component "OG Rail"
equation "tape_thickness = 0.7 mm"
equation "stiffness = 1.0"
equation "d154 = tape_thickness + 2 * printer_tolerance"
equation "d198 = ( 35 / 2 ) * 1 mm"
equation "d209 = 1.4 mm * stiffness"
equation "d224 = foam_thickness"
equation "d228 = rail_angle"
equation "rail_angle = 14 deg"
equation "foam_thickness = 6 mm"
equation "tape_width = 8 mm"
equation "d241 = tape_width + cassette_wall_thickness * 2 + 2 * printer_tolerance"
equation "d243 = -cassette_wall_thickness"
equation "d245 = -cassette_wall_thickness"
equation "rail_length = 200 mm"
equation "d255 = rail_length / 2"
equation "d264 = -rail_divider_thickness"
equation "rail_dividers = 2"
equation "rail_divider_thickness = 1.8 mm"
equation "d272 = rail_dividers + 2"
equation "d274 = -rail_length + 3 * rail_divider_thickness"
equation "d276 = -2 * rail_divider_thickness"
equation "d280 = -2 * rail_divider_thickness"
equation "d282 = ( 4 * 0.4 ) * 1 mm"
equation "d294 = -printer_tolerance"
equation "d295 = -printer_tolerance"
equation "printer_tolerance = 0.2 mm"
equation "cassette_wall_thickness = 0.9 mm"
equation "d198_1 = ( 35 / 2 ) * 1 mm"
equation "d209_1 = 1.4 mm * stiffness"
equation "d241_1 = 3 * cassette_wall_thickness + ( 2 * 4 ) * 1 mm"
equation "d305 = cassette_wall_thickness"
equation "d308 = -cassette_wall_thickness"
equation "d317 = ( 0.4 * 3 ) * 1 mm"
named bodies: "Cassette", "OG Rail Body", "Divider", "Divider (1)", "Divider (2)", "Divider (3)", "OG Rail Lid"
